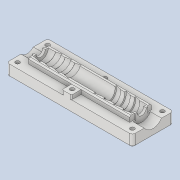
# Autodesk Inventor part: MoldeB_leveled
Saved by Autodesk Inventor 2020.4 (Build 244396000, 396)
## iProperties
Part Number: MoldeB_leveled
Material: Acetalharz, weiß
Document SubType Name: Modeling
Designer: rYan
Mass: 7.87255 g
Surface Area: 45.3022 cm^2
Volume: 5.5246 cm^3
Density: 1.425 g/cm^3
Appearance: Glatt - weiß
Author: rYan
Autodesk Inventor part; units mm, degrees
ref_plane "YZ Plane" through (0, 0, 0) normal (1, 0, 0) x (0, 1, 0)
ref_plane "XZ Plane" through (0, 0, 0) normal (0, 1, 0) x (-1, 0, 0)
ref_plane "XY Plane" through (0, 0, 0) normal (0, 0, 1) x (1, 0, 0)
sketch "Skizze1" plane through (0, 0, 0) normal (1, 0, 0) x (0, 1, 0)
  circle A0 centre (0, 0) radius 3
  circle A1 centre (0, 0) radius 5.5
  dimension "d0" = 6
  dimension "d1" = 11
  constraints: 2 centre point, 2 coincident
  measures "d0" diameter of A0
  measures "d1" diameter of A1
extrude "Extrusion1" add sketch "Skizze1" along normal blind 36
sketch "Skizze3" plane through (0, 0, 0) normal (0, 1, 0) x (-1, 0, 0)
  line L0 (-36, 5.5) -> (-32, 5.5)
  line L1 (-32, 5.5) -> (-32.1763, 6.5)
  line L2 (-32.1763, 6.5) -> (-36, 5.6)
  line L3 (-36, 5.6) -> (-36, 5.5)
  line L4 (-36, 5.5) -> (-36, -5.5) construction
  line L5 (0, -5.5) -> (0, 5.5) construction
  point P0 (0, 0)
  dimension "d16" = 4
  dimension "d17" = 80
  dimension "d18" = 1
  dimension "d19" = 0.1
  constraints: 8 end point, 1 horizontal, 1 vertical
  measures "d16" distance of L0.start L0.end
  measures "d17" angle of L1 L0
  measures "d18" distance from line of L0 L1.end
  measures "d19" distance of L2.end L0.start
coil "Spirale1" sketch "Skizze3" operation add axis through (-10, 0, 0) along (-1, 0, 0) pitch 7 turns 3.5 hand left
mirror "Spiegeln1" about plane through (0, 0, 0) normal (1, 0, 0) of "Extrusion1", "Spirale1"
sketch "Sketch7" plane through (36, 0, 0) normal (1, 0, 0) x (0, 0, -1)
  line L0 (-12, -15) -> (12, -15)
  line L1 (12, -15) -> (12, 15)
  line L2 (12, 15) -> (-12, 15)
  line L3 (-12, 15) -> (-12, -15)
  line L4 (-12, -15) -> (12, 15) construction
  line L5 (12, -15) -> (-12, 15) construction
  point P0 (0, 0)
  dimension "d39" = 24
  dimension "d40" = 30
  constraints: 12 end point, 2 midpoint, 2 parallel, 1 horizontal, 1 perpendicular
  measures "d39" distance of L1.end L2.end
  measures "d40" distance of L0.end L1.end
extrude "Extrusion5" add sketch "Sketch7" along normal blind 10 and the other way blind 82 separate body
sketch "Sketch8" plane through (-46, 0, 0) normal (-1, 0, 0) x (0, 0, -1)
  circle A0 centre (0, 0) radius 3.5
  dimension "d34" = 7
  constraints: 1 centre point, 1 coincident
  measures "d34" diameter of A0
extrude "Extrusion6" add sketch "Sketch8" against normal up to surface (92 mm away) separate body
combine bodies "Combine1" operation type subtract main body 2 bodies to subtract 1 3
sketch "Sketch9" plane through (-46, -15, 12) normal (0, 0, 1) x (1, 0, 0)
  line L0 (0, 0) -> (92, 0) projected
  line L1 (92, 30) -> (92, 0) projected
  line L2 (0, 30) -> (92, 30) projected
  line L3 (0, 0) -> (0, 30) projected
  point P0 (46, 15)
extrude "Extrusion7" cut sketch "Sketch9" against normal blind 12 bodies 2
sketch "Sketch10" plane through (-46, -15, 0) normal (0, 0, 1) x (1, 0, 0)
  line L0 (9, 7) -> (83, 7)
  line L1 (83, 7) -> (83, 23)
  line L2 (83, 23) -> (9, 23)
  line L3 (9, 23) -> (9, 7)
  line L4 (9, 7) -> (83, 23) construction
  line L5 (83, 7) -> (9, 23) construction
  line L6 (82, 11.5) -> (92, 11.5) projected
  line L7 (92, 18.5) -> (92, 11.5) projected
  line L8 (92, 18.5) -> (82, 18.5) projected
  line L9 (82, 18.5) -> (82, 11.5) projected
  line L10 (0, 11.5) -> (10, 11.5) projected
  line L11 (10, 11.5) -> (10, 18.5) projected
  line L12 (10, 18.5) -> (0, 18.5) projected
  line L13 (0, 11.5) -> (0, 18.5) projected
  line L14 (6.5, 4.5) -> (85.5, 4.5)
  line L15 (85.5, 4.5) -> (85.5, 25.5)
  line L16 (85.5, 25.5) -> (6.5, 25.5)
  line L17 (6.5, 25.5) -> (6.5, 4.5)
  line L18 (6.5, 4.5) -> (85.5, 25.5) construction
  line L19 (85.5, 4.5) -> (6.5, 25.5) construction
  line L20 (0, 11.5) -> (10, 11.5) projected
  line L21 (0, 0) -> (0, 11.5) projected
  line L22 (92, 0) -> (0, 0) projected
  line L23 (92, 11.5) -> (92, 0) projected
  line L24 (82, 11.5) -> (92, 11.5) projected
  line L25 (82, 9.5) -> (82, 11.5) projected
  line L26 (80.25, 9.5) -> (82, 9.5) projected
  line L27 (73.25, 9.5) -> (76.25, 9.5) projected
  line L28 (66.25, 9.5) -> (69.25, 9.5) projected
  line L29 (59.25, 9.5) -> (62.25, 9.5) projected
  line L30 (36.75, 9.5) -> (55.25, 9.5) projected
  line L31 (29.75, 9.5) -> (32.75, 9.5) projected
  line L32 (22.75, 9.5) -> (25.75, 9.5) projected
  line L33 (15.75, 9.5) -> (18.75, 9.5) projected
  line L34 (10, 9.5) -> (11.75, 9.5) projected
  line L35 (10, 11.5) -> (10, 9.5) projected
  line L36 (10, 18.5) -> (0, 18.5) projected
  line L37 (10, 20.5) -> (10, 18.5) projected
  line L38 (15.25, 20.5) -> (10, 20.5) projected
  line L39 (22.25, 20.5) -> (19.25, 20.5) projected
  line L40 (29.25, 20.5) -> (26.25, 20.5) projected
  line L41 (58.75, 20.5) -> (33.25, 20.5) projected
  line L42 (65.75, 20.5) -> (62.75, 20.5) projected
  line L43 (72.75, 20.5) -> (69.75, 20.5) projected
  line L44 (82, 20.5) -> (76.75, 20.5) projected
  line L45 (82, 18.5) -> (82, 20.5) projected
  line L46 (92, 18.5) -> (82, 18.5) projected
  line L47 (92, 30) -> (92, 18.5) projected
  line L48 (0, 30) -> (92, 30) projected
  line L49 (0, 18.5) -> (0, 30) projected
  line L50 (0, 30) -> (0, 0) projected
  line L51 (9, 19.5) -> (0, 19.5)
  line L52 (0, 19.5) -> (0, 10.5)
  line L53 (0, 10.5) -> (9, 10.5)
  line L54 (6.5, 10.5) -> (6.5, 19.5)
  line L55 (82, 19.5) -> (92, 19.5)
  line L56 (92, 19.5) -> (92, 10.5)
  line L57 (92, 10.5) -> (82, 10.5)
  line L58 (82, 10.5) -> (82, 19.5)
  point P0 (46, 15)
  point P1 (9, 18.5)
  point P2 (83, 18.5)
  point P3 (83, 11.5)
  point P4 (9, 11.5)
  point P5 (6.5, 10.5)
  point P6 (6.5, 11.5)
  point P7 (6.5, 18.5)
  point P8 (83, 19.5)
  point P9 (83, 10.5)
  dimension "d43" = 74
  dimension "d44" = 16
  dimension "d45" = 79
  dimension "d46" = 21
  dimension "d63" = 1
  dimension "d64" = 1
  dimension "d65" = 1
  dimension "d66" = 1
  constraints: 40 end point, 14 vertical alignment, 8 parallel, 7 point on line, 5 midpoint, 4 horizontal, 4 perpendicular, 28 other
  measures "d43" distance of L2.end L1.end
  measures "d44" distance of L1.end L0.end
  measures "d45" distance of L16.end L15.end
  measures "d46" distance of L15.end L14.end
  measures "d63" distance between parallel lines of L12 L51
  measures "d64" distance between parallel lines of L10 L53
  measures "d65" distance between parallel lines of L55 L8
  measures "d66" distance between parallel lines of L6 L57
extrude "Extrusion8" cut sketch "Sketch10" against normal blind 4 contours L0 L1 L57 L15 L14 L17 L53 L3 | L17 L14 L15 L57 L23 L22 L21 L53 | L51 L17 L16 L15 L55 L1 L2 L3 | L51 L49 L48 L47 L55 L15 L16 L17 bodies 2
sketch "Sketch11" plane through (46, 15, -12) normal (0, 0, -1) x (-1, 0, 0)
  line L0 (0, 0) -> (92, 0) projected
  line L1 (0, -30) -> (0, 0) projected
  line L2 (92, -30) -> (0, -30) projected
  line L3 (92, 0) -> (92, -30) projected
  circle A0 centre (4, -4) radius 1.5
  circle A1 centre (4, -26) radius 1.5
  circle A2 centre (88, -4) radius 1.5
  circle A3 centre (88, -26) radius 1.5
  circle A4 centre (48, -26) radius 1.5
  circle A5 centre (46, -4) radius 1.5
  point P0 (46, -15)
  dimension "d49" = 3
  dimension "d50" = 3
  dimension "d51" = 3
  dimension "d52" = 3
  dimension "d53" = 4
  dimension "d54" = 4
  dimension "d55" = 4
  dimension "d56" = 4
  dimension "d57" = 4
  dimension "d58" = 4
  dimension "d59" = 4
  dimension "d60" = 4
  dimension "d75" = 3
  dimension "d76" = 3
  dimension "d77" = 4
  dimension "d78" = 46
  dimension "d79" = 4
  dimension "d80" = 44
  constraints: 6 centre point
  measures "d49" diameter of A0
  measures "d50" diameter of A1
  measures "d51" diameter of A2
  measures "d52" diameter of A3
  measures "d53" distance from line of L1 A0.centre
  measures "d54" distance from line of L0 A0.centre
  measures "d55" distance from line of L2 A1.centre
  measures "d56" distance from line of L1 A1.centre
  measures "d57" distance from line of A3.centre L2
  measures "d58" distance from line of L3 A3.centre
  measures "d59" distance from line of L3 A2.centre
  measures "d60" distance from line of L0 A2.centre
  measures "d75" diameter of A4
  measures "d76" diameter of A5
  measures "d77" distance from line of A5.centre L0
  measures "d78" distance from line of L3 A5.centre
  measures "d79" distance from line of L2 A4.centre
  measures "d80" distance from line of L3 A4.centre
extrude "Extrusion9" cut sketch "Sketch11" against normal up to surface (8 mm away) contours A0 | A1 | A2 | A3 | A4 | A5 bodies 2
sketch "Sketch12" plane through (-46, 0, 0) normal (-1, 0, 0) x (0, 0, 1)
  circle A0 centre (0, 0) radius 3
  arc A1 (0, 3.5) -> (0, -3.5) centre (0, 0) ccw projected
  line L0 (0, 3.5) -> (0, 3)
  line L1 (0, -3.5) -> (0, -3)
  dimension "d67" = 6
  constraints: 4 end point, 2 point on circle, 1 centre point, 1 coincident, 1 point on line, 1 vertical
  measures "d67" diameter of A0
extrude "Extrusion10" add sketch "Sketch12" against normal up to surface (10 mm away) contours A0 L1 A1 L0 bodies 2
sketch "Sketch13" plane through (46, 0, 0) normal (1, 0, 0) x (0, 0, -1)
  line L0 (4, 15) -> (4, 4.5) projected
  line L1 (4, 4.5) -> (0, 4.5) projected
  line L2 (0, 4.5) -> (0, 3.5) projected
  arc A0 (0, -3.5) -> (0, 3.5) centre (0, 0) ccw projected
  line L3 (0, -3.5) -> (0, -4.5) projected
  line L4 (0, -4.5) -> (4, -4.5) projected
  line L5 (4, -4.5) -> (4, -15) projected
  line L6 (4, -15) -> (12, -15) projected
  line L7 (12, -15) -> (12, 15) projected
  line L8 (12, 15) -> (4, 15) projected
  line L9 (0, -3) -> (0, -5.5) projected
  arc A1 (0, -5.5) -> (0, 5.5) centre (0, 0) ccw projected
  line L10 (0, 5.5) -> (0, 3) projected
  arc A2 (0, -3) -> (0, 3) centre (0, 0) ccw projected
  point P0 (0, -3.5)
  point P1 (0, 3.5)
extrude "Extrusion11" add sketch "Sketch13" against normal up to surface (10 mm away) contours A0 L9 A2 L10 bodies 2
chamfer "Chamfer2" distance 1 angle 45 2 edges at (0, -8, 0) (0, 8, 0)
sketch "Sketch14" plane through (46, 15, -12) normal (0, 0, -1) x (-1, 0, 0)
  circle A0 centre (4, -26) radius 1.5 projected
  circle A1 centre (48, -26) radius 1.5 projected
  circle A2 centre (88, -26) radius 1.5 projected
  circle A3 centre (88, -4) radius 1.5 projected
  circle A4 centre (46, -4) radius 1.5 projected
  circle A5 centre (4, -4) radius 1.5 projected
  circle A6 centre (4, -4) radius 2.75
  circle A7 centre (46, -4) radius 2.75
  circle A8 centre (88, -4) radius 2.75
  circle A9 centre (88, -26) radius 2.75
  circle A10 centre (48, -26) radius 2.75
  circle A11 centre (4, -26) radius 1.5 projected
  circle A12 centre (4, -26) radius 2.75
  point P0 (46, -15)
  dimension "d81" = 5.5
  dimension "d82" = 5.5
  dimension "d83" = 5.5
  dimension "d84" = 5.5
  dimension "d85" = 5.5
  dimension "d86" = 5.5
  constraints: 6 centre point, 6 coincident
  measures "d81" diameter of A6
  measures "d82" diameter of A7
  measures "d83" diameter of A8
  measures "d84" diameter of A9
  measures "d85" diameter of A10
  measures "d86" diameter of A12
extrude "Extrusion12" cut sketch "Sketch14" against normal blind 5 contours A0 | A1 | A2 | A3 | A4 | A5 | A6 | A7 | A8 | A9 | A10 | A12 bodies 2
fillet "Fillet1" radius 2 4 edges at (46, -15, -8) (46, 15, -8) (-46, 15, -8) (-46, -15, -8)
fillet "Fillet1" radius 0.5 4 edges at (0, 15, -12) (46, 0, -12) (0, -15, -12) (-46, 0, -12)
sketch "Sketch15" plane through (-36, 0, 0) normal (1, 0, 0) x (0, 0, -1)
  arc A0 (0, -3) -> (0, 3) centre (0, 0) ccw projected
  circle A1 centre (0, 0) radius 3.25
  line L0 (0, -4.5) -> (0, -3) projected
  line L1 (0, 3) -> (0, 4.5) projected
  point P0 (0, -3.25)
  point P1 (0, 3.25)
  dimension "d91" = 6.5
  constraints: 1 centre point, 1 coincident
  measures "d91" diameter of A1
extrude "Extrusion13" cut sketch "Sketch15" along normal blind 74.1 and the other way blind 2.1 contours A0 L1 A1 L0 picked at (3.0688, 0) bodies 2
fillet "Fillet2" radius 1 4 edges at (-46, -4.5, -2) (-46, 4.5, -2) (46, -4.5, -2) (46, 4.5, -2)
sketch "Sketch16" plane through (-38.1, 0, 0) normal (1, 0, 0) x (0, 0, -1)
  arc A0 (0, -3) -> (0, 3) centre (0, 0) ccw projected
  circle A1 centre (0, 0) radius 6
  dimension "d97" = 12
  constraints: 1 centre point, 1 coincident
  measures "d97" diameter of A1
extrude "Extrusion14" cut sketch "Sketch16" along normal blind 0.2 and the other way blind 7.9 bodies 2
sketch "Sketch17" plane through (38.1, 0, 0) normal (-1, 0, 0) x (0, 0, 1)
  arc A0 (0, 3) -> (0, -3) centre (0, 0) ccw projected
  circle A1 centre (0, 0) radius 7.5
  dimension "d102" = 15
  constraints: 1 centre point, 1 coincident
  measures "d102" diameter of A1
extrude "Extrusion15" cut sketch "Sketch17" along normal blind 0.2 and the other way blind 7.9 bodies 2
sketch "Sketch19" plane through (-46, -15, -4) normal (0, 0, 1) x (1, 0, 0)
  line L0 (9, 7) -> (83, 7) projected
  circle A0 centre (44, 4) radius 1.5 projected
  line L1 (40.5, 0) -> (47.5, 0)
  line L2 (47.5, 0) -> (47.5, 7)
  line L3 (47.5, 6.9) -> (40.5, 6.9)
  line L4 (40.5, 7) -> (40.5, 0)
  line L5 (40.5, 0) -> (47.5, 6.9) construction
  line L6 (47.5, 0) -> (40.5, 6.9) construction
  line L7 (90, 0) -> (2, 0) projected
  point P0 (46, 15)
  point P1 (44, 3.45)
  dimension "d116" = 0
  dimension "d117" = 0
  dimension "d118" = 7
  constraints: 12 end point, 4 point on line, 2 midpoint, 2 parallel, 1 horizontal, 1 perpendicular
  measures "d116" horizontal distance of A0.centre point (44, 3.45)
  measures "d117" distance between parallel lines of L7 L1
  measures "d118" distance between parallel lines of L2 L4
extrude "Extrusion17" add sketch "Sketch19" along normal blind 3 bodies 2
fillet "Fillet3" radius 1 2 edges at (1.5, -15, -2.5) (-5.5, -15, -2.5)
body "Solid2"
